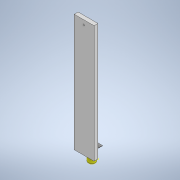
# Autodesk Inventor part: spray
Saved by Autodesk Inventor 2022 (Build 260153000, 153)
## iProperties
Created: 2022-08-22
Part Number: spray
Material: Generic
Document SubType Name: Modeling
Designer: Sachin
Density: 1 g/cm^3
Appearance: Default
Author: Sachin
Autodesk Inventor part; units mm, degrees
ref_plane "YZ Plane" through (0, 0, 0) normal (1, 0, 0) x (0, 1, 0)
ref_plane "XZ Plane" through (0, 0, 0) normal (0, 1, 0) x (-1, 0, 0)
ref_plane "XY Plane" through (0, 0, 0) normal (0, 0, 1) x (1, 0, 0)
sketch "Sketch1" plane through (0, 0, 0) normal (0, 0, 1) x (1, 0, 0)
  line L0 (0, 0) -> (-25.4, 0)
  line L1 (-25.4, 0) -> (-25.4, 150)
  line L2 (-25.4, 150) -> (0, 150)
  line L3 (0, 150) -> (0, 0)
  dimension "d0" = 25.4
  dimension "d1" = 150
  constraints: 8 end point, 2 parallel, 1 horizontal, 1 perpendicular
  measures "d0" distance of L1.end L2.end
  measures "d1" distance of L0.end L1.end
extrude "Extrusion1" add sketch "Sketch1" along normal blind 5
sketch "Sketch2" plane through (0, 0, 0) normal (0, 0, -1) x (-1, 0, 0)
  point P0 (0, 0)
sketch "Sketch3" plane through (0, 0, 0) normal (0, 0, -1) x (-1, 0, 0)
  line L0 (4.1948, 7.7945) -> (22.3514, 7.7945)
  line L1 (22.3514, 7.7945) -> (22.3514, 7.4454)
  line L2 (22.3514, 7.4454) -> (4.1948, 7.4454)
  line L3 (4.1948, 7.4454) -> (4.1948, 7.7945)
  point P0 (0, 0)
  constraints: 8 end point, 2 parallel, 1 horizontal, 1 perpendicular
extrude "Extrusion2" add sketch "Sketch3" along normal blind 10
sketch "Sketch4" plane through (-22.3514, 7.4454, 0) normal (0, -1, 0) x (1, 0, 0)
  circle A0 centre (9.6514, -4.8899) radius 4.6183
  point P0 (22.3514, 0)
  constraints: 1 centre point
extrude "Extrusion3" add sketch "Sketch4" along normal blind 20
fillet "Fillet1" radius 2 1 edges at (-17.3183, -12.5546, -4.8899)
sketch "Sketch5" plane through (-12.7, -12.5546, -4.8899) normal (0, -1, 0) x (1, 0, 0)
  circle A0 centre (0, 0) radius 2.6183 projected
  circle A1 centre (0, 0) radius 0.7983
  point P0 (12.7, 4.8899)
  constraints: 1 centre point, 1 coincident
extrude "Extrusion4" cut sketch "Sketch5" against normal blind 20 contours A1
sketch "Sketch6" plane through (0, 0, 5) normal (0, 0, 1) x (1, 0, 0)
  circle A0 centre (-13.1019, 144.2767) radius 1
  point P0 (0, 0)
  dimension "d11" = 2
  constraints: 1 centre point
  measures "d11" diameter of A0
extrude "Extrusion5" cut sketch "Sketch6" against normal blind 20
sketch "Sketch7" plane through (-22.3514, 7.7945, 0) normal (0, 1, 0) x (1, 0, 0)
  circle A0 centre (9.6514, 4.8899) radius 0.7983 projected
  circle A1 centre (9.6514, 4.8899) radius 2.5276
  point P0 (22.3514, 0)
  constraints: 1 centre point, 1 coincident
extrude "Extrusion6" add sketch "Sketch7" along normal blind 120
body "Solid1"
